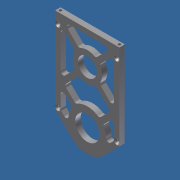
# Autodesk Inventor part: Lower box side plate
Saved by Autodesk Inventor 2012 (Build 160160000, 160)
## iProperties
Created: 2012-07-07
Part Number: Lower box side plate
Material: Default
Document SubType Name: Modeling
Designer: Bryce
Density: 1 g/cm^3
Author: Bryce
Autodesk Inventor part; units mm, degrees
ref_plane "YZ Plane" through (0, 0, 0) normal (1, 0, 0) x (0, 1, 0)
ref_plane "XZ Plane" through (0, 0, 0) normal (0, 1, 0) x (-1, 0, 0)
ref_plane "XY Plane" through (0, 0, 0) normal (0, 0, 1) x (1, 0, 0)
sketch "Sketch1" plane through (0, 0, 0) normal (0, 0, 1) x (1, 0, 0)
  line L0 (-38.1, 50.8) -> (38.1, 50.8)
  line L1 (38.1, 50.8) -> (38.1, -50.8)
  line L2 (-38.1, -50.8) -> (-38.1, 50.8)
  circle A0 centre (0, 11.7) radius 11.1125
  line L3 (-38.1, -50.8) -> (0, -88.9)
  line L4 (0, -88.9) -> (38.1, -50.8)
  circle A1 centre (0, -50.8) radius 14.2875
  point P0 (0, 0)
  point P1 (-34.925, -47.625)
  point P2 (34.925, -47.625)
  point P3 (-34.925, 38.1)
  point P4 (34.925, 38.1)
  dimension "d0" = 76.2
  dimension "d1" = 38.1
  dimension "d2" = 101.6
  dimension "d3" = 50.8
  dimension "d4" = 101.6
  dimension "d5" = 38.1
  dimension "d6" = 38.1
  dimension "d7" = 28.575
  dimension "d8" = 38.1
  dimension "d9" = 38.1
  dimension "d10" = 22.225
  dimension "d11" = 38.1
  dimension "d13" = 3.175
  dimension "d14" = 12.7
  dimension "d15" = 3.175
  dimension "d16" = 3.175
  dimension "d17" = 3.175
  dimension "d18" = 3.175
  dimension "d31" = 3.175
  dimension "d32" = 12.7
  dimension "d88" = 62.5
  constraints: 10 end point, 2 centre point, 1 horizontal, 1 parallel, 1 perpendicular
  measures "d0" distance of L0.start L0.end
  measures "d1" distance from line of L2 point (0, 0)
  measures "d2" distance of L0.end L1.end
  measures "d3" distance from line of L0 point (0, 0)
  measures "d4" distance of L2.start L0.start
  measures "d5" horizontal distance of L2.start L3.end
  measures "d6" horizontal distance of L3.end L1.end
  measures "d7" diameter of A1
  measures "d8" distance from line of L1 A1.centre
  measures "d9" distance of L3.end A1.centre
  measures "d10" diameter of A0
  measures "d11" distance from line of L1 A0.centre
  measures "d13" distance from line of L2 point (-34.925, 38.1)
  measures "d14" distance from line of L0 point (-34.925, 38.1)
  measures "d15" horizontal distance of L2.start point (-34.925, -47.625)
  measures "d16" distance from line of L2 point (-34.925, -47.625)
  measures "d17" horizontal distance of L1.end point (34.925, -47.625)
  measures "d18" distance from line of L1 point (34.925, -47.625)
  measures "d31" distance from line of L1 point (34.925, 38.1)
  measures "d32" distance from line of L0 point (34.925, 38.1)
  measures "d88" distance of A1.centre A0.centre
extrude "Extrusion1" add sketch "Sketch1" against normal blind 6.35
fillet "Fillet1" radius 26.9494 1 edges at (0, -88.9, -3.175)
sketch "Sketch2" plane through (0, 0, 0) normal (0, 0, 1) x (1, 0, 0)
  line L0 (-38.1, 50.8) -> (38.1, 50.8) projected
  line L1 (-38.1, -50.8) -> (-38.1, 50.8) projected
  line L2 (38.1, -50.8) -> (19.0561, -69.8439) projected
  line L3 (38.1, 50.8) -> (38.1, -50.8) projected
  line L4 (-19.0561, -69.8439) -> (-38.1, -50.8) projected
  circle A0 centre (0, -50.8) radius 14.2875 projected
  line L5 (-31.75, 44.45) -> (31.75, 44.45)
  line L6 (31.75, 44.45) -> (31.75, -48.1697)
  line L7 (-31.75, -48.1697) -> (-31.75, 44.45)
  line L8 (-31.75, -48.1697) -> (-20.4747, -59.445)
  line L9 (31.75, -48.1697) -> (20.4747, -59.445)
  arc A1 (20.4747, -59.445) -> (-20.4747, -59.445) centre (0, -50.8) ccw
  arc A2 (9.897, 26.0871) -> (-9.897, 26.0871) centre (0, 11.7) ccw
  arc A3 (14.3871, 1.803) -> (14.3871, 21.597) centre (0, 11.7) ccw
  arc A4 (-9.897, -2.6871) -> (9.897, -2.6871) centre (0, 11.7) ccw
  arc A5 (-14.3871, 21.597) -> (-14.3871, 1.803) centre (0, 11.7) ccw
  line L10 (0, 11.7) -> (-31.75, 43.45) construction
  line L11 (-31.75, 43.45) -> (0, 11.7) construction
  line L12 (0, 11.7) -> (31.75, 43.45) construction
  line L13 (0, 11.7) -> (-31.75, -20.05) construction
  line L14 (0, 11.7) -> (31.75, -20.05) construction
  line L15 (-31.75, 38.9599) -> (-14.3871, 21.597) construction
  line L16 (-14.3871, 21.597) -> (-31.75, 38.9599)
  line L17 (-28.2599, 44.45) -> (-9.897, 26.0871)
  line L18 (28.2599, 44.45) -> (9.897, 26.0871)
  line L19 (31.75, 38.9599) -> (14.3871, 21.597)
  line L20 (31.75, -15.5599) -> (14.3871, 1.803)
  line L21 (14.3871, 1.803) -> (31.75, -15.5599)
  line L22 (31.75, -24.5401) -> (9.897, -2.6871)
  line L23 (-31.75, -24.5401) -> (-9.897, -2.6871)
  line L24 (-31.75, -15.5599) -> (-14.3871, 1.803)
  line L25 (-31.75, -20.05) -> (0, -50.8) construction
  line L26 (0, -50.8) -> (31.75, -20.05) construction
  line L27 (-18.0398, -37.8186) -> (-31.75, -24.5401)
  line L28 (31.75, -24.5401) -> (18.396, -38.3285)
  line L29 (27.2599, -20.05) -> (14.1094, -33.6281)
  line L30 (-27.2593, -20.0494) -> (-13.6325, -33.247)
  point P0 (38.1, -47.625)
  point P1 (38.1, 41.275)
  point P2 (25.4, 50.8)
  point P3 (-25.4, 50.8)
  point P4 (-38.1, 41.275)
  point P5 (-38.1, -47.625)
  point P6 (-34.925, 38.1)
  point P7 (-34.925, -47.625)
  point P8 (34.925, 38.1)
  point P9 (34.925, -47.625)
  dimension "d92" = 12.7
  dimension "d93" = 3.175
  dimension "d96" = 85.725
  dimension "d99" = 69.85
  dimension "d106" = 6.35
  dimension "d107" = 6.35
  dimension "d108" = 6.35
  dimension "d109" = 6.35
  dimension "d110" = 6.35
  dimension "d111" = 22.225
  dimension "d112" = 17.4625
  dimension "d113" = 6.35
  dimension "d114" = 3.175
  dimension "d115" = 6.35
  dimension "d116" = 3.175
  dimension "d117" = 6.35
  dimension "d118" = 3.175
  dimension "d119" = 6.35
  dimension "d120" = 3.175
  dimension "d121" = 6.35
  dimension "d122" = 6.3492
  constraints: 52 end point, 14 point on circle, 14 point on line, 10 perpendicular, 9 parallel, 5 centre point, 5 coincident, 4 collinear, 3 concentric, 2 horizontal, 1 vertical, 3 other
  measures "d92" distance from line of L0 point (-34.925, 38.1)
  measures "d93" distance from line of L1 point (-34.925, 38.1)
  measures "d96" distance of point (-34.925, 38.1) point (-34.925, -47.625)
  measures "d99" distance of point (-34.925, 38.1) point (34.925, 38.1)
  measures "d106" distance between parallel lines of L4 L8
  measures "d107" distance between parallel lines of L2 L9
  measures "d108" distance between parallel lines of L7 L1
  measures "d109" distance between parallel lines of L5 L0
  measures "d110" distance between parallel lines of L3 L6
  measures "d111" radius of A1
  measures "d112" radius of A2
  measures "d113" distance between parallel lines of L15 L17
  measures "d114" distance between parallel lines of L15 L10
  measures "d115" distance between parallel lines of L19 L18
  measures "d116" distance between parallel lines of L12 L18
  measures "d117" distance between parallel lines of L22 L20
  measures "d118" distance between parallel lines of L14 L21
  measures "d119" distance between parallel lines of L23 L24
  measures "d120" distance between parallel lines of L23 L13
  measures "d121" distance between parallel lines of L27 L30
  measures "d122" distance between parallel lines of L28 L29
hole "Hole3" at (-34.925, -47.625, 0) at (34.925, -47.625, 0) at (-34.925, 38.1, 0) at (34.925, 38.1, 0) direction (0, 0, -1) diameter 3.175 end through all countersink diameter 6.35 countersink angle 82
sketch "Sketch3" plane through (-38.1, 50.8, 0) normal (0, 1, 0) x (1, 0, 0)
  line L0 (0, 0) -> (0, 6.35) projected
  line L1 (0, 0) -> (76.2, 0) projected
  line L2 (76.2, 0) -> (76.2, 6.35) projected
  point P0 (38.1, 0)
  point P1 (3.175, 3.175)
  point P2 (73.025, 3.175)
  dimension "d77" = 3.175
  dimension "d78" = 3.175
  dimension "d79" = 3.175
  constraints: 1 horizontal alignment
  measures "d77" distance from line of L1 point (3.175, 3.175)
  measures "d78" distance from line of L0 point (3.175, 3.175)
  measures "d79" distance from line of L2 point (73.025, 3.175)
hole "Hole4" at (-34.925, 50.8, -3.175) at (34.925, 50.8, -3.175) direction (0, -1, 0) diameter 3.175 depth 9.525 tip angle 118
extrude "Extrusion4" cut sketch "Sketch2" against normal blind 25.4 contours L5 L18 A2 L17 | L16 A5 L24 L7 | L27 A1 L8 L7 | L6 L20 A3 L19 | L23 A4 L22 L29 A1 L30 | L6 L9 A1 L28
fillet "Fillet4" radius 3.175 26 edges at (-28.2599, 44.45, -3.175) (-9.897, 26.0871, -3.175) (28.2599, 44.45, -3.175) (9.897, 26.0871, -3.175) (14.3871, 21.597, -3.175) (-14.3871, 1.803, -3.175) (14.3871, 1.803, -3.175) (31.75, 38.9599, -3.175) (-14.3871, 21.597, -3.175) (-31.75, 38.9599, -3.175) (-31.75, -15.5599, -3.175) (31.75, -15.5599, -3.175) (9.897, -2.6871, -3.175) (-9.897, -2.6871, -3.175) (-27.2593, -20.0494, -3.175) (27.2599, -20.05, -3.175) (14.1094, -33.6281, -3.175) (-13.6325, -33.247, -3.175) (-31.75, -24.5401, -3.175) (-18.0398, -37.8186, -3.175) (-31.75, -48.1697, -3.175) (-20.4747, -59.445, -3.175) (20.4747, -59.445, -3.175) (31.75, -48.1697, -3.175) (31.75, -24.5401, -3.175) (18.396, -38.3285, -3.175)
equation "\"d108\" = d106"
equation "\"d109\" = d108"
equation "\"d110\" = d109"
body "Solid1"
